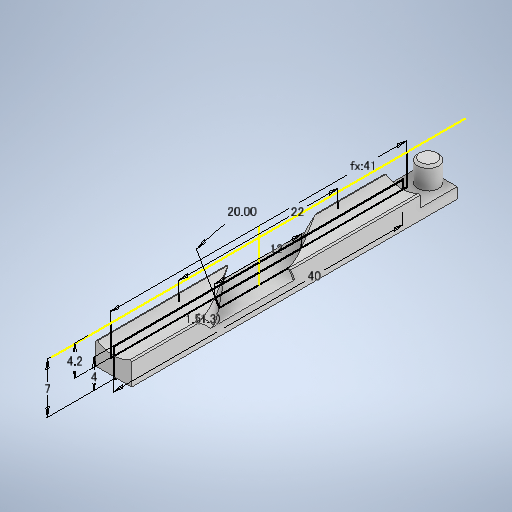
# Autodesk Inventor part: SwitchLeverUnit_Slider
Saved by Autodesk Inventor 2025.1 (Build 291241000, 241)
## iProperties
Created: 2025-03-08
Part Number: SwitchLeverUnit_Slider
Material: 一般
Document SubType Name: Modeling
Designer: kumagai
Density: 1 g/cm^3
Appearance: 既定
Author: kumagai
Autodesk Inventor part; units mm, degrees
ref_plane "YZ Plane" through (0, 0, 0) normal (1, 0, 0) x (0, 1, 0)
ref_plane "XZ Plane" through (0, 0, 0) normal (0, 1, 0) x (-1, 0, 0)
ref_plane "XY Plane" through (0, 0, 0) normal (0, 0, 1) x (1, 0, 0)
sketch "ProfileSketch" plane through (0, 0, 0) normal (1, 0, 0) x (0, 1, 0)
  line L0 (0, 28.7) -> (0, -28.7) projected
  line L1 (-8.4, 0) -> (1.4, 0) projected
  line L2 (-3, 20) -> (-7, 20)
  line L3 (-7, 20) -> (-7, -20)
  line L4 (-7, -20) -> (-3, -20)
  line L5 (-3, -20) -> (-3, 20)
  line L6 (-4.2, 6) -> (-5.7, 5.454)
  line L7 (-5.7, 5.454) -> (-5.7, -5.454)
  line L8 (-5.7, -5.454) -> (-4.2, -6)
  line L9 (0, 20.5) -> (-4.2, 20.5)
  line L10 (-4.2, 20.5) -> (-4.2, -20.5)
  line L11 (-4.2, -20.5) -> (0, -20.5)
  line L12 (-2.1072, 11) -> (-1.3293, 11)
  line L13 (-1.9893, -11) -> (-1.3293, -11)
  dimension "d1" = 40
  dimension "d2" = 41
  dimension "d3" = 4.2
  dimension "d4" = 7
  dimension "d5" = 4
  dimension "d6" = 1.5
  dimension "d7" = 20
  dimension "d8" = 12
  dimension "d28" = 22
  dimension "d29" = 1.3
  constraints: 24 end point, 4 point on line, 1 vertical, 4 other
  measures "d1" distance between parallel lines of L4 L2
  measures "d2" distance between parallel lines of L11 L9
  measures "d3" distance between parallel lines of L10 L0
  measures "d4" distance between parallel lines of L0 L3
  measures "d5" distance between parallel lines of L3 L5
  measures "d6" distance between parallel lines of L10 L7
  measures "d7" angle of L1 L6
  measures "d8" distance of L8.end L6.start
  measures "d28" distance between parallel lines of L13 L12
  measures "d29" distance between parallel lines of L3 L7
extrude "SliderBody" add sketch "ProfileSketch" along normal mid plane 5 contours L5 L4 L10 L1 | L1 L10 L2 L5 | L10 L6 L7 L1 L3 L2 | L10 L8 L7 L1 | L1 L7 L6 L10 | L4 L3 L1 L7 L8 L10
revolve "BodyTop" cut sketch "ProfileSketch" angle 360 about axis through (0, 0, 0) along (0, 0, -1) contours L0 L1 L5 L2 L10 L9 | L0 L11 L10 L4 L5 L1 | L5 L4 L10 L1 | L1 L10 L2 L5
coil "Screw1" sketch "ProfileSketch" operation cut axis through (0, 0, 0) along (0, 0, -1) pitch 45 turns 0.333333 hand right contours L10 L8 L7 L1 | L1 L7 L6 L10
coil "Screw2" sketch "ProfileSketch" operation cut axis through (0, 0, 0) along (0, 0, 1) pitch 45 turns 0.333333 hand right contours L10 L8 L7 L1 | L1 L7 L6 L10
sketch "ConnectingPinSketch" plane through (0, 0, 0) normal (0, 1, 0) x (-1, 0, 0)
  line L0 (0, -29.4) -> (0, 4.9) projected
  line L1 (-3.5, 0) -> (3.5, 0) projected
  circle A0 centre (0, -23.5) radius 1.45
  line L2 (2.5, -25) -> (-2.5, -25)
  line L3 (-2.5, -25) -> (-2.5, -19.9)
  line L4 (-2.5, -19.9) -> (2.5, -19.9)
  line L5 (2.5, -19.9) -> (2.5, -25)
  point P0 (0, 0)
  dimension "d30" = 2.9
  dimension "d31" = 23.5
  dimension "d32" = 1.5
  dimension "d33" = 3.6
  dimension "d34" = 5
  constraints: 8 end point, 2 horizontal, 1 centre point, 1 point on line, 1 other
  measures "d30" diameter of A0
  measures "d31" distance from line of L1 A0.centre
  measures "d32" distance from line of A0.centre L2
  measures "d33" distance from line of A0.centre L4
  measures "d34" distance between parallel lines of L3 L5
extrude "CP_Cut" cut sketch "ConnectingPinSketch" against normal through all contours L2 L3 L4 L0 A0 | L0 A0 L4 L5 L2
extrude "CP_Body" add sketch "ConnectingPinSketch" along normal blind 1.8 from surface at -7
extrude "CP_Pin" add sketch "ConnectingPinSketch" along normal blind 3 from surface at -5.2 contours A0 L0 | L0 A0
chamfer "CP_Chamfer" distance 0.3 angle 45 1 edges at (1.45, -2.2, -23.5)
chamfer "SliderBodyChamfer" distance 0.3 angle 45 12 edges at (2.5, -4.2047, 9.5901) (-2.5, -4.2085, 1.908) (2.5, -4.2085, -1.908) (-2.5, -4.2047, -9.5901) (2.5, -3.3749, 15.2831) (-2.5, -3.3749, 10.7169) (-2.5, -3.3749, -15.2331) (2.5, -3.3749, -10.6669) (2.5, -7, -2.5) (-2.5, -7, -2.5) (0, -7, 20) (0, -7, -25)
